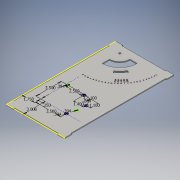
# Autodesk Inventor part: main board
Saved by Autodesk Inventor 2016 SP2 (Build 200236200, 236)
## iProperties
Created: 2017-09-03
Part Number: main board
Material: Generic
Document SubType Name: Modeling
Designer: Kartikye
Density: 1 g/cm^3
Appearance: Default
Author: Kartikye
Autodesk Inventor part; units mm, degrees
ref_plane "YZ Plane" through (0, 0, 0) normal (1, 0, 0) x (0, 1, 0)
ref_plane "XZ Plane" through (0, 0, 0) normal (0, 1, 0) x (-1, 0, 0)
ref_plane "XY Plane" through (0, 0, 0) normal (0, 0, 1) x (1, 0, 0)
sketch "Sketch1" plane through (0, 0, 0) normal (0, 1, 0) x (-1, 0, 0)
  line L0 (0, 0) -> (203.2, 0)
  line L1 (203.2, 0) -> (203.2, -381)
  line L2 (203.2, -381) -> (0, -381)
  line L3 (0, -381) -> (0, 0)
  dimension "d0" = 203.2
  dimension "d1" = 381
  constraints: 8 end point, 2 parallel, 1 horizontal, 1 perpendicular
  measures "d0" distance of L1.end L2.end
  measures "d1" distance of L0.end L1.end
extrude "Extrusion1" add sketch "Sketch1" along normal blind 3.175
sketch "Sketch2" plane through (0, 3.175, 0) normal (0, 1, 0) x (1, 0, 0)
  circle A0 centre (-158.75, 351.3667) radius 3.175
  line L0 (-203.2, 381) -> (-203.2, 0) projected
  line L1 (0, 381) -> (-203.2, 381) projected
  point P0 (0, 0)
  dimension "d4" = 6.35
  dimension "d5" = 44.45
  dimension "d6" = 29.6333
  constraints: 1 centre point
  measures "d4" diameter of A0
  measures "d5" distance from line of L0 A0.centre
  measures "d6" distance from line of L1 A0.centre
extrude "Extrusion2" cut sketch "Sketch2" against normal blind 3.175
sketch "Sketch3" plane through (0, 3.175, 0) normal (0, 1, 0) x (1, 0, 0)
  line L0 (-203.2, 381) -> (-203.2, 0) projected
  line L1 (0, 381) -> (-203.2, 381) projected
  line L2 (-203.2, 381) -> (0, 381) projected
  line L3 (-203.2, 0) -> (-203.2, 381) projected
  circle A0 centre (-158.75, 351.3667) radius 3.175 projected
  line L4 (-158.75, 351.3667) -> (-158.75, 197.5357) construction
  arc A1 (-158.75, 224.3667) -> (-31.75, 351.3667) centre (-158.75, 351.3667) ccw construction
  line L5 (-31.75, 351.3667) -> (-158.75, 351.3667) construction
  line L6 (-56.0048, 276.7179) -> (-158.75, 351.3667) construction
  line L7 (-77.7972, 253.5115) -> (-158.75, 351.3667) construction
  line L8 (-60.8948, 270.4138) -> (-158.75, 351.3667) construction
  line L9 (-66.171, 264.4292) -> (-158.75, 351.3667) construction
  line L10 (-71.8125, 258.7877) -> (-158.75, 351.3667) construction
  line L11 (-57.9661, 280.1712) -> (-65.672, 285.7698)
  line L12 (-65.672, 285.7698) -> (-67.5382, 283.2012)
  line L13 (-67.5382, 283.2012) -> (-59.8323, 277.6025)
  line L14 (-59.8323, 277.6025) -> (-57.9661, 280.1712)
  arc A2 (-77.7972, 253.5115) -> (-56.0048, 276.7179) centre (-158.75, 351.3667) ccw
  circle A3 centre (-67.9205, 285.3752) radius 1.27
  line L15 (-64.6418, 271.5575) -> (-62.6185, 274.0043)
  line L16 (-62.6185, 274.0043) -> (-69.959, 280.0742)
  line L17 (-71.9823, 277.6274) -> (-64.6418, 271.5575)
  line L18 (-69.959, 280.0742) -> (-71.9823, 277.6274)
  circle A4 centre (-72.2278, 279.8211) radius 1.27
  arc A5 (-166.6967, 224.6155) -> (-31.9989, 343.4199) centre (-158.75, 351.3667) ccw construction
  line L19 (-69.8201, 265.8253) -> (-67.6477, 268.1407)
  line L20 (-67.6477, 268.1407) -> (-74.5939, 274.658)
  line L21 (-76.7664, 272.3426) -> (-69.8201, 265.8253)
  line L22 (-74.5939, 274.658) -> (-76.7664, 272.3426)
  circle A6 centre (-76.8742, 274.5473) radius 1.27
  arc A7 (-174.6123, 225.3612) -> (-32.7445, 335.5043) centre (-158.75, 351.3667) ccw construction
  line L23 (-75.3469, 260.4283) -> (-73.0339, 262.6033)
  line L24 (-73.0339, 262.6033) -> (-79.5587, 269.5425)
  line L25 (-81.8718, 267.3675) -> (-75.3469, 260.4283)
  line L26 (-79.5587, 269.5425) -> (-81.8718, 267.3675)
  circle A8 centre (-81.8414, 269.5747) radius 1.27
  arc A9 (-182.4658, 226.6006) -> (-33.984, 327.6509) centre (-158.75, 351.3667) ccw construction
  line L27 (-81.2006, 255.3878) -> (-78.756, 257.4137)
  line L28 (-78.756, 257.4137) -> (-84.8339, 264.7476)
  line L29 (-87.2785, 262.7216) -> (-81.2006, 255.3878)
  line L30 (-84.8339, 264.7476) -> (-87.2785, 262.7216)
  circle A10 centre (-87.1101, 264.9226) radius 1.27
  arc A11 (-190.2263, 228.3291) -> (-35.7124, 319.8904) centre (-158.75, 351.3667) ccw construction
  line L31 (-28.9364, 348.5365) -> (-28.9236, 349.6672)
  line L32 (-28.9236, 349.6672) -> (-31.7607, 349.6994)
  line L33 (-31.7607, 349.6994) -> (-31.7555, 350.1627)
  line L34 (-31.7555, 350.1627) -> (-28.9183, 350.1305)
  line L35 (-28.9183, 350.1305) -> (-28.9056, 351.2481)
  line L36 (-28.9056, 351.2481) -> (-28.568, 351.2442)
  line L37 (-28.568, 351.2442) -> (-28.5988, 348.5327)
  line L38 (-28.5988, 348.5327) -> (-28.9364, 348.5365)
  line L39 (-32.0967, 341.9) -> (-32.0669, 342.3623)
  line L40 (-32.0669, 342.3623) -> (-30.6668, 342.272)
  line L41 (-30.6668, 342.272) -> (-30.5595, 343.9359)
  line L42 (-30.5595, 343.9359) -> (-31.9596, 344.0262)
  line L43 (-31.9596, 344.0262) -> (-31.9298, 344.4885)
  line L44 (-31.9298, 344.4885) -> (-28.7613, 344.2842)
  line L45 (-28.7613, 344.2842) -> (-28.7912, 343.8219)
  line L46 (-28.7912, 343.8219) -> (-30.2226, 343.9142)
  line L47 (-30.2226, 343.9142) -> (-30.3298, 342.2503)
  line L48 (-30.3298, 342.2503) -> (-28.8984, 342.158)
  line L49 (-28.8984, 342.158) -> (-28.9283, 341.6957)
  line L50 (-28.9283, 341.6957) -> (-32.0967, 341.9)
  spline S0 degree 2 poles (-32.0758, 334.4167) (-31.8629, 334.3895) (-31.53, 334.682) (-31.375, 335.0897) knots 0 0 0 1 2 2 2
  spline S1 degree 2 poles (-31.375, 335.0897) (-31.1895, 335.5911) (-30.653, 336.1136) (-30.3025, 336.0688) knots 0 0 0 1 2 2 2
  spline S2 degree 2 poles (-30.3025, 336.0688) (-29.9338, 336.0217) (-29.5205, 335.3329) (-29.5842, 334.8344) knots 0 0 0 1 2 2 2
  spline S3 degree 2 poles (-29.5842, 334.8344) (-29.6529, 334.297) (-30.2979, 333.7303) (-30.6731, 333.7888) knots 0 0 0 1 2 2 2
  line L51 (-30.6731, 333.7888) -> (-30.6854, 333.7957)
  line L52 (-30.6854, 333.7957) -> (-30.6293, 334.2344)
  spline S4 degree 2 poles (-30.6293, 334.2344) (-30.3619, 334.2003) (-29.9596, 334.5605) (-29.9191, 334.8772) knots 0 0 0 1 2 2 2
  spline S5 degree 2 poles (-29.9191, 334.8772) (-29.878, 335.1992) (-30.1224, 335.5787) (-30.356, 335.6086) knots 0 0 0 1 2 2 2
  spline S6 degree 2 poles (-30.356, 335.6086) (-30.5612, 335.6348) (-30.8819, 335.2932) (-31.0398, 334.8833) knots 0 0 0 1 2 2 2
  spline S7 degree 2 poles (-31.0398, 334.8833) (-31.2302, 334.3851) (-31.7792, 333.9091) (-32.1323, 333.9542) knots 0 0 0 1 2 2 2
  spline S8 degree 2 poles (-32.1323, 333.9542) (-32.5114, 334.0026) (-32.8905, 334.7108) (-32.8242, 335.2301) knots 0 0 0 1 2 2 2
  spline S9 degree 2 poles (-32.8242, 335.2301) (-32.7611, 335.7234) (-32.1557, 336.4139) (-31.7289, 336.3461) knots 0 0 0 1 2 2 2
  line L53 (-31.7289, 336.3461) -> (-31.7163, 336.3419)
  line L54 (-31.7163, 336.3419) -> (-31.7727, 335.9005)
  spline S10 degree 2 poles (-31.7727, 335.9005) (-32.0687, 335.9383) (-32.4527, 335.494) (-32.4918, 335.1876) knots 0 0 0 1 2 2 2
  spline S11 degree 2 poles (-32.4918, 335.1876) (-32.5337, 334.8605) (-32.3095, 334.4465) (-32.0758, 334.4167) knots 0 0 0 1 2 2 2
  line L55 (-32.4656, 327.2848) -> (-31.047, 326.1028)
  line L56 (-31.047, 326.1028) -> (-31.1465, 325.5809)
  line L57 (-31.1465, 325.5809) -> (-32.9418, 327.1491)
  line L58 (-32.9418, 327.1491) -> (-34.0397, 327.3585)
  line L59 (-34.0397, 327.3585) -> (-33.9534, 327.811)
  line L60 (-33.9534, 327.811) -> (-32.8247, 327.5957)
  line L61 (-32.8247, 327.5957) -> (-30.6125, 328.3809)
  line L62 (-30.6125, 328.3809) -> (-30.7115, 327.8615)
  line L63 (-30.7115, 327.8615) -> (-32.4656, 327.2848)
  line L64 (-34.3099, 320.2407) -> (-35.5423, 320.5558)
  line L65 (-35.5423, 320.5558) -> (-35.4275, 321.0046)
  line L66 (-35.4275, 321.0046) -> (-32.3515, 320.2182)
  line L67 (-32.3515, 320.2182) -> (-32.6763, 318.9477)
  spline S12 degree 2 poles (-32.6763, 318.9477) (-32.8125, 318.4151) (-33.4707, 317.9539) (-33.8841, 318.0596) knots 0 0 0 1 2 2 2
  spline S13 degree 2 poles (-33.8841, 318.0596) (-34.3025, 318.1666) (-34.6561, 318.8865) (-34.5199, 319.419) knots 0 0 0 1 2 2 2
  line L68 (-34.5199, 319.419) -> (-34.3099, 320.2407)
  line L69 (-33.9827, 320.157) -> (-34.1928, 319.3354)
  spline S14 degree 2 poles (-34.1928, 319.3354) (-34.279, 318.9981) (-34.0299, 318.5778) (-33.7737, 318.5123) knots 0 0 0 1 2 2 2
  spline S15 degree 2 poles (-33.7737, 318.5123) (-33.5176, 318.4468) (-33.0897, 318.694) (-33.0035, 319.0313) knots 0 0 0 1 2 2 2
  line L70 (-33.0035, 319.0313) -> (-32.7934, 319.8529)
  line L71 (-32.7934, 319.8529) -> (-33.9827, 320.157)
  spline S16 degree 2 poles (-37.1074, 310.5406) (-37.6602, 310.7196) (-38.1497, 311.6979) (-37.9578, 312.2906) knots 0 0 0 1 2 2 2
  spline S17 degree 2 poles (-37.9578, 312.2906) (-37.7732, 312.8608) (-36.8122, 313.3393) (-36.2593, 313.1604) knots 0 0 0 1 2 2 2
  line L72 (-36.2593, 313.1604) -> (-35.7214, 312.9862)
  spline S18 degree 2 poles (-35.7214, 312.9862) (-35.1711, 312.8081) (-34.6678, 311.8556) (-34.8525, 311.2853) knots 0 0 0 1 2 2 2
  spline S19 degree 2 poles (-34.8525, 311.2853) (-35.0443, 310.6926) (-36.0167, 310.1875) (-36.5695, 310.3665) knots 0 0 0 1 2 2 2
  line L73 (-36.5695, 310.3665) -> (-37.1074, 310.5406)
  spline S20 degree 2 poles (-36.421, 310.8082) (-36.0077, 310.6743) (-35.3208, 310.9857) (-35.1886, 311.3941) knots 0 0 0 1 2 2 2
  spline S21 degree 2 poles (-35.1886, 311.3941) (-35.0637, 311.7801) (-35.4458, 312.41) (-35.8592, 312.5439) knots 0 0 0 1 2 2 2
  line L74 (-35.8592, 312.5439) -> (-36.402, 312.7196)
  spline S22 degree 2 poles (-36.402, 312.7196) (-36.8204, 312.855) (-37.4991, 312.5685) (-37.6241, 312.1825) knots 0 0 0 1 2 2 2
  spline S23 degree 2 poles (-37.6241, 312.1825) (-37.7571, 311.7717) (-37.3848, 311.1201) (-36.9639, 310.9839) knots 0 0 0 1 2 2 2
  line L75 (-36.9639, 310.9839) -> (-36.421, 310.8082)
  line L76 (-39.9728, 302.4007) -> (-39.4456, 303.7065)
  line L77 (-39.4456, 303.7065) -> (-40.499, 304.1317)
  line L78 (-40.499, 304.1317) -> (-41.1163, 302.6026)
  line L79 (-41.1163, 302.6026) -> (-41.427, 302.7281)
  line L80 (-41.427, 302.7281) -> (-40.6363, 304.6868)
  line L81 (-40.6363, 304.6868) -> (-37.6921, 303.4982)
  line L82 (-37.6921, 303.4982) -> (-38.4731, 301.5638)
  line L83 (-38.4731, 301.5638) -> (-38.7862, 301.6902)
  line L84 (-38.7862, 301.6902) -> (-38.1787, 303.195)
  line L85 (-38.1787, 303.195) -> (-39.1325, 303.5801)
  line L86 (-39.1325, 303.5801) -> (-39.6597, 302.2743)
  line L87 (-39.6597, 302.2743) -> (-39.9728, 302.4007)
  line L88 (-42.5334, 296.8254) -> (-43.7767, 297.4169)
  line L89 (-43.7767, 297.4169) -> (-43.5777, 297.8352)
  line L90 (-43.5777, 297.8352) -> (-40.7129, 296.4725)
  line L91 (-40.7129, 296.4725) -> (-41.2166, 295.4136)
  spline S24 degree 2 poles (-41.2166, 295.4136) (-41.4583, 294.9054) (-42.1319, 294.5678) (-42.529, 294.7567) knots 0 0 0 1 2 2 2
  spline S25 degree 2 poles (-42.529, 294.7567) (-42.7489, 294.8613) (-42.957, 295.2646) (-42.9403, 295.5495) knots 0 0 0 1 2 2 2
  spline S26 degree 2 poles (-42.9403, 295.5495) (-43.1398, 295.3313) (-43.5882, 295.2721) (-43.8435, 295.3936) knots 0 0 0 1 2 2 2
  line L92 (-43.8435, 295.3936) -> (-44.1129, 295.5218)
  spline S27 degree 2 poles (-44.1129, 295.5218) (-44.2477, 295.5858) (-44.4908, 295.6232) (-44.5952, 295.5743) knots 0 0 0 1 2 2 2
  line L93 (-44.5952, 295.5743) -> (-44.6424, 295.5968)
  line L94 (-44.6424, 295.5968) -> (-44.4367, 296.0294)
  spline S28 degree 2 poles (-44.4367, 296.0294) (-44.3311, 296.0806) (-44.0487, 296.0042) (-43.9092, 295.9379) knots 0 0 0 1 2 2 2
  line L95 (-43.9092, 295.9379) -> (-43.6492, 295.8142)
  spline S29 degree 2 poles (-43.6492, 295.8142) (-43.4152, 295.7029) (-42.9921, 295.8611) (-42.8752, 296.1069) knots 0 0 0 1 2 2 2
  line L96 (-42.8752, 296.1069) -> (-42.5334, 296.8254)
  line L97 (-42.2285, 296.6804) -> (-42.5129, 296.0824)
  spline S30 degree 2 poles (-42.5129, 296.0824) (-42.6816, 295.7278) (-42.5806, 295.2943) (-42.3253, 295.1728) knots 0 0 0 1 2 2 2
  spline S31 degree 2 poles (-42.3253, 295.1728) (-42.0842, 295.0582) (-41.6721, 295.236) (-41.5192, 295.5575) knots 0 0 0 1 2 2 2
  line L98 (-41.5192, 295.5575) -> (-41.2144, 296.198)
  line L99 (-41.2144, 296.198) -> (-42.2285, 296.6804)
  line L100 (-47.0424, 290.2452) -> (-47.8506, 288.7808)
  line L101 (-47.8506, 288.7808) -> (-48.1439, 288.9427)
  line L102 (-48.1439, 288.9427) -> (-47.1119, 290.8127)
  line L103 (-47.1119, 290.8127) -> (-44.3321, 289.2786)
  line L104 (-44.3321, 289.2786) -> (-44.556, 288.873)
  line L105 (-44.556, 288.873) -> (-47.0424, 290.2452)
  spline S32 degree 2 poles (-51.1536, 281.4624) (-51.3657, 281.5971) (-51.6558, 281.9704) (-51.7289, 282.1874) knots 0 0 0 1 2 2 2
  line L106 (-51.7289, 282.1874) -> (-52.3914, 282.0034)
  line L107 (-52.3914, 282.0034) -> (-52.4567, 282.4231)
  line L108 (-52.4567, 282.4231) -> (-51.7863, 282.6145)
  spline S33 degree 2 poles (-51.7863, 282.6145) (-51.7797, 282.8056) (-51.656, 283.186) (-51.5396, 283.3694) knots 0 0 0 1 2 2 2
  spline S34 degree 2 poles (-51.5396, 283.3694) (-51.2183, 283.8754) (-50.1682, 284.0985) (-49.6776, 283.787) knots 0 0 0 1 2 2 2
  line L109 (-49.6776, 283.787) -> (-49.2003, 283.484)
  spline S35 degree 2 poles (-49.2003, 283.484) (-48.712, 283.1739) (-48.4628, 282.1258) (-48.7841, 281.6198) knots 0 0 0 1 2 2 2
  spline S36 degree 2 poles (-48.7841, 281.6198) (-49.118, 281.0939) (-50.1858, 280.8479) (-50.6763, 281.1594) knots 0 0 0 1 2 2 2
  line L110 (-50.6763, 281.1594) -> (-51.1536, 281.4624)
  spline S37 degree 2 poles (-50.4222, 281.5499) (-50.0554, 281.317) (-49.3125, 281.4468) (-49.0824, 281.8092) knots 0 0 0 1 2 2 2
  spline S38 degree 2 poles (-49.0824, 281.8092) (-48.8649, 282.1517) (-49.0775, 282.8572) (-49.4443, 283.0901) knots 0 0 0 1 2 2 2
  line L111 (-49.4443, 283.0901) -> (-49.926, 283.3959)
  spline S39 degree 2 poles (-49.926, 283.3959) (-50.2972, 283.6316) (-51.026, 283.5239) (-51.2435, 283.1814) knots 0 0 0 1 2 2 2
  spline S40 degree 2 poles (-51.2435, 283.1814) (-51.475, 282.8168) (-51.2773, 282.0929) (-50.9039, 281.8558) knots 0 0 0 1 2 2 2
  line L112 (-50.9039, 281.8558) -> (-50.4222, 281.5499)
  line L113 (-55.7542, 275.674) -> (-54.9953, 276.7177)
  line L114 (-54.9953, 276.7177) -> (-55.4757, 277.4456)
  line L115 (-55.4757, 277.4456) -> (-55.1971, 277.8288)
  line L116 (-55.1971, 277.8288) -> (-53.3557, 274.9624)
  line L117 (-53.3557, 274.9624) -> (-53.5897, 274.6406)
  line L118 (-53.5897, 274.6406) -> (-56.8703, 275.5276)
  line L119 (-56.8703, 275.5276) -> (-56.5917, 275.9108)
  line L120 (-56.5917, 275.9108) -> (-55.7542, 275.674)
  line L121 (-54.7817, 276.3973) -> (-55.3835, 275.5695)
  line L122 (-55.3835, 275.5695) -> (-53.9902, 275.1713)
  line L123 (-53.9902, 275.1713) -> (-53.981, 275.184)
  line L124 (-53.981, 275.184) -> (-54.7817, 276.3973)
  line L125 (-61.2151, 270.0279) -> (-60.9174, 270.3862)
  line L126 (-60.9174, 270.3862) -> (-58.4753, 268.3572)
  line L127 (-58.4753, 268.3572) -> (-58.773, 267.9989)
  line L128 (-58.773, 267.9989) -> (-61.2151, 270.0279)
  line L129 (-66.6794, 262.4131) -> (-66.6925, 262.4183)
  spline S41 degree 2 poles (-66.6925, 262.4183) (-67.023, 262.7202) (-66.9798, 263.6379) (-66.5858, 264.0543) knots 0 0 0 1 2 2 2
  spline S42 degree 2 poles (-66.5858, 264.0543) (-66.1863, 264.4763) (-65.1293, 264.485) (-64.7035, 264.082) knots 0 0 0 1 2 2 2
  line L130 (-64.7035, 264.082) -> (-64.2929, 263.6934)
  spline S43 degree 2 poles (-64.2929, 263.6934) (-63.867, 263.2904) (-63.8157, 262.2327) (-64.2151, 261.8107) knots 0 0 0 1 2 2 2
  spline S44 degree 2 poles (-64.2151, 261.8107) (-64.6163, 261.3867) (-65.504, 261.2827) (-65.8408, 261.6122) knots 0 0 0 1 2 2 2
  line L131 (-65.8408, 261.6122) -> (-65.8467, 261.625)
  line L132 (-65.8467, 261.625) -> (-65.5409, 261.9482)
  spline S45 degree 2 poles (-65.5409, 261.9482) (-65.2994, 261.7197) (-64.7266, 261.7614) (-64.4603, 262.0428) knots 0 0 0 1 2 2 2
  spline S46 degree 2 poles (-64.4603, 262.0428) (-64.1941, 262.3241) (-64.2957, 263.0582) (-64.6075, 263.3533) knots 0 0 0 1 2 2 2
  line L133 (-64.6075, 263.3533) -> (-65.022, 263.7455)
  spline S47 degree 2 poles (-65.022, 263.7455) (-65.3375, 264.0442) (-66.0761, 264.1053) (-66.3424, 263.824) knots 0 0 0 1 2 2 2
  spline S48 degree 2 poles (-66.3424, 263.824) (-66.6087, 263.5426) (-66.6207, 262.9702) (-66.3736, 262.7363) knots 0 0 0 1 2 2 2
  line L134 (-66.3736, 262.7363) -> (-66.6794, 262.4131)
  spline S49 degree 2 poles (-72.7661, 257.3144) (-72.7957, 257.5265) (-72.5551, 258.1552) (-72.2028, 258.4835) knots 0 0 0 1 2 2 2
  spline S50 degree 2 poles (-72.2028, 258.4835) (-71.7681, 258.8887) (-70.7033, 258.8865) (-70.3107, 258.4652) knots 0 0 0 1 2 2 2
  line L135 (-70.3107, 258.4652) -> (-69.8645, 257.9866)
  spline S51 degree 2 poles (-69.8645, 257.9866) (-69.4701, 257.5634) (-69.5215, 256.5207) (-69.9542, 256.1174) knots 0 0 0 1 2 2 2
  spline S52 degree 2 poles (-69.9542, 256.1174) (-70.3735, 255.7265) (-71.2417, 255.6866) (-71.534, 256.0117) knots 0 0 0 1 2 2 2
  line L136 (-71.534, 256.0117) -> (-71.5391, 256.0249)
  line L137 (-71.5391, 256.0249) -> (-71.2136, 256.3283)
  spline S53 degree 2 poles (-71.2136, 256.3283) (-71.0155, 256.1158) (-70.4563, 256.1109) (-70.1845, 256.3644) knots 0 0 0 1 2 2 2
  spline S54 degree 2 poles (-70.1845, 256.3644) (-69.8973, 256.6321) (-69.9162, 257.3587) (-70.2017, 257.6651) knots 0 0 0 1 2 2 2
  line L138 (-70.2017, 257.6651) -> (-70.6515, 258.1476)
  spline S55 degree 2 poles (-70.6515, 258.1476) (-70.9388, 258.4558) (-71.6833, 258.5097) (-71.9743, 258.2385) knots 0 0 0 1 2 2 2
  spline S56 degree 2 poles (-71.9743, 258.2385) (-72.1964, 258.0314) (-72.3569, 257.6815) (-72.3522, 257.5498) knots 0 0 0 1 2 2 2
  line L139 (-72.3522, 257.5498) -> (-71.865, 257.0271)
  line L140 (-71.865, 257.0271) -> (-71.2963, 257.5572)
  line L141 (-71.2963, 257.5572) -> (-71.0679, 257.3121)
  line L142 (-71.0679, 257.3121) -> (-71.9754, 256.4662)
  line L143 (-71.9754, 256.4662) -> (-72.7661, 257.3144)
  line L144 (-76.3224, 250.6123) -> (-76.6799, 250.3177)
  line L145 (-76.6799, 250.3177) -> (-78.1132, 252.0568)
  spline S57 degree 2 poles (-78.1132, 252.0568) (-78.3962, 252.4002) (-78.279, 253.1718) (-77.9215, 253.4664) knots 0 0 0 1 2 2 2
  spline S58 degree 2 poles (-77.9215, 253.4664) (-77.5559, 253.7677) (-76.831, 253.7647) (-76.5577, 253.4167) knots 0 0 0 1 2 2 2
  line L146 (-76.5577, 253.4167) -> (-76.5535, 253.4033)
  line L147 (-76.5535, 253.4033) -> (-76.8968, 253.1203)
  spline S59 degree 2 poles (-76.8968, 253.1203) (-77.0849, 253.3485) (-77.4963, 253.3826) (-77.7084, 253.2078) knots 0 0 0 1 2 2 2
  spline S60 degree 2 poles (-77.7084, 253.2078) (-77.9064, 253.0447) (-77.9388, 252.5737) (-77.7557, 252.3515) knots 0 0 0 1 2 2 2
  line L148 (-77.7557, 252.3515) -> (-76.3224, 250.6123)
  line L149 (-83.023, 248.0395) -> (-83.3131, 248.3434)
  line L150 (-83.3131, 248.3434) -> (-83.3274, 248.3363)
  line L151 (-83.3274, 248.3363) -> (-83.1461, 247.9507)
  line L152 (-83.1461, 247.9507) -> (-82.4261, 245.9141)
  line L153 (-82.4261, 245.9141) -> (-82.7955, 245.6477)
  line L154 (-82.7955, 245.6477) -> (-84.5049, 246.9709)
  line L155 (-84.5049, 246.9709) -> (-84.8202, 247.2695)
  line L156 (-84.8202, 247.2695) -> (-84.8308, 247.2618)
  line L157 (-84.8308, 247.2618) -> (-84.6322, 246.879)
  line L158 (-84.6322, 246.879) -> (-83.8189, 244.9098)
  line L159 (-83.8189, 244.9098) -> (-84.2265, 244.6158)
  line L160 (-84.2265, 244.6158) -> (-85.4105, 247.6764)
  line L161 (-85.4105, 247.6764) -> (-85.0751, 247.9183)
  line L162 (-85.0751, 247.9183) -> (-83.2313, 246.5339)
  line L163 (-83.2313, 246.5339) -> (-83.022, 246.3331)
  line L164 (-83.022, 246.3331) -> (-83.0114, 246.3408)
  line L165 (-83.0114, 246.3408) -> (-83.1379, 246.6013)
  line L166 (-83.1379, 246.6013) -> (-83.8628, 248.7925)
  line L167 (-83.8628, 248.7925) -> (-83.5253, 249.0359)
  line L168 (-83.5253, 249.0359) -> (-80.9973, 246.9444)
  line L169 (-80.9973, 246.9444) -> (-81.4049, 246.6505)
  line L170 (-81.4049, 246.6505) -> (-83.023, 248.0395)
  line L171 (-89.8994, 240.8822) -> (-91.033, 242.6615)
  spline S61 degree 2 poles (-91.033, 242.6615) (-91.3143, 243.103) (-91.0112, 243.9913) (-90.5211, 244.3035) knots 0 0 0 1 2 2 2
  spline S62 degree 2 poles (-90.5211, 244.3035) (-90.0509, 244.6031) (-89.134, 244.4889) (-88.8542, 244.0496) knots 0 0 0 1 2 2 2
  line L172 (-88.8542, 244.0496) -> (-87.7206, 242.2703)
  line L173 (-87.7206, 242.2703) -> (-88.1135, 242.02)
  line L174 (-88.1135, 242.02) -> (-89.2471, 243.7993)
  spline S63 degree 2 poles (-89.2471, 243.7993) (-89.4426, 244.1061) (-90.0409, 244.2122) (-90.3411, 244.0209) knots 0 0 0 1 2 2 2
  spline S64 degree 2 poles (-90.3411, 244.0209) (-90.659, 243.8184) (-90.8378, 243.2173) (-90.6423, 242.9104) knots 0 0 0 1 2 2 2
  line L175 (-90.6423, 242.9104) -> (-89.5087, 241.1312)
  line L176 (-89.5087, 241.1312) -> (-89.8994, 240.8822)
  line L177 (-96.3627, 240.7396) -> (-94.83, 237.9591)
  line L178 (-94.83, 237.9591) -> (-95.7744, 237.4385)
  spline S65 degree 2 poles (-95.7744, 237.4385) (-96.3635, 237.1138) (-97.4489, 237.3912) (-97.7408, 237.9207) knots 0 0 0 1 2 2 2
  line L179 (-97.7408, 237.9207) -> (-97.9506, 238.3012)
  spline S66 degree 2 poles (-97.9506, 238.3012) (-98.2437, 238.833) (-97.8962, 239.8943) (-97.3071, 240.2191) knots 0 0 0 1 2 2 2
  line L180 (-97.3071, 240.2191) -> (-96.3627, 240.7396)
  line L181 (-95.3987, 238.0311) -> (-96.6067, 240.2226)
  line L182 (-96.6067, 240.2226) -> (-97.1453, 239.9256)
  spline S67 degree 2 poles (-97.1453, 239.9256) (-97.5625, 239.6957) (-97.7634, 238.9214) (-97.5448, 238.5249) knots 0 0 0 1 2 2 2
  line L183 (-97.5448, 238.5249) -> (-97.3325, 238.1398)
  spline S68 degree 2 poles (-97.3325, 238.1398) (-97.1165, 237.7478) (-96.3546, 237.5042) (-95.9374, 237.7342) knots 0 0 0 1 2 2 2
  line L184 (-95.9374, 237.7342) -> (-95.3987, 238.0311)
  line L185 (-103.5851, 235.3824) -> (-103.3129, 235.5109)
  line L186 (-103.3129, 235.5109) -> (-103.9253, 236.808)
  line L187 (-103.9253, 236.808) -> (-103.5063, 237.0058)
  line L188 (-103.5063, 237.0058) -> (-102.1508, 234.1347)
  line L189 (-102.1508, 234.1347) -> (-102.5698, 233.9369)
  line L190 (-102.5698, 233.9369) -> (-103.1698, 235.2079)
  line L191 (-103.1698, 235.2079) -> (-103.3994, 235.0995)
  line L192 (-103.3994, 235.0995) -> (-103.9497, 233.2854)
  line L193 (-103.9497, 233.2854) -> (-104.4231, 233.0619)
  line L194 (-104.4231, 233.0619) -> (-104.4323, 233.0691)
  line L195 (-104.4323, 233.0691) -> (-103.8169, 235.0211)
  line L196 (-103.8169, 235.0211) -> (-105.8688, 235.8788)
  line L197 (-105.8688, 235.8788) -> (-105.8685, 235.8905)
  line L198 (-105.8685, 235.8905) -> (-105.3596, 236.1308)
  line L199 (-105.3596, 236.1308) -> (-103.5851, 235.3824)
  line L200 (-111.0187, 231.59) -> (-111.3044, 230.1433)
  line L201 (-111.3044, 230.1433) -> (-111.8247, 229.936)
  line L202 (-111.8247, 229.936) -> (-111.3966, 231.8028)
  line L203 (-111.3966, 231.8028) -> (-113.0221, 232.8766)
  line L204 (-113.0221, 232.8766) -> (-112.509, 233.0811)
  line L205 (-112.509, 233.0811) -> (-111.2794, 232.2158)
  line L206 (-111.2794, 232.2158) -> (-110.9797, 233.6906)
  line L207 (-110.9797, 233.6906) -> (-110.4569, 233.899)
  line L208 (-110.4569, 233.899) -> (-110.8981, 232.0015)
  line L209 (-110.8981, 232.0015) -> (-109.3033, 230.9409)
  line L210 (-109.3033, 230.9409) -> (-109.8212, 230.7345)
  line L211 (-109.8212, 230.7345) -> (-111.0187, 231.59)
  line L212 (-118.0337, 231.0651) -> (-117.0427, 228.0487)
  line L213 (-117.0427, 228.0487) -> (-118.1045, 227.6999)
  spline S69 degree 2 poles (-118.1045, 227.6999) (-118.6168, 227.5316) (-119.3277, 227.7499) (-119.4617, 228.1577) knots 0 0 0 1 2 2 2
  spline S70 degree 2 poles (-119.4617, 228.1577) (-119.5262, 228.3541) (-119.3664, 228.7483) (-119.1787, 228.8981) knots 0 0 0 1 2 2 2
  spline S71 degree 2 poles (-119.1787, 228.8981) (-119.5134, 228.835) (-120.0277, 229.1426) (-120.1241, 229.4361) knots 0 0 0 1 2 2 2
  spline S72 degree 2 poles (-120.1241, 229.4361) (-120.2597, 229.8488) (-119.8216, 230.4777) (-119.3243, 230.6411) knots 0 0 0 1 2 2 2
  line L214 (-119.3243, 230.6411) -> (-118.0337, 231.0651)
  line L215 (-118.009, 229.5056) -> (-118.3693, 230.6022)
  line L216 (-118.3693, 230.6022) -> (-119.2197, 230.3228)
  spline S73 degree 2 poles (-119.2197, 230.3228) (-119.5231, 230.2231) (-119.7656, 229.8376) (-119.6823, 229.584) knots 0 0 0 1 2 2 2
  spline S74 degree 2 poles (-119.6823, 229.584) (-119.5998, 229.3328) (-119.1586, 229.1389) (-118.8669, 229.2237) knots 0 0 0 1 2 2 2
  line L217 (-118.8669, 229.2237) -> (-118.837, 229.2335)
  line L218 (-118.837, 229.2335) -> (-118.009, 229.5056)
  line L219 (-117.9044, 229.1873) -> (-118.6181, 228.9528)
  spline S75 degree 2 poles (-118.6181, 228.9528) (-118.8643, 228.8719) (-119.0926, 228.5186) (-119.0191, 228.2948) knots 0 0 0 1 2 2 2
  spline S76 degree 2 poles (-119.0191, 228.2948) (-118.939, 228.0511) (-118.5232, 227.9177) (-118.2099, 228.0207) knots 0 0 0 1 2 2 2
  line L220 (-118.2099, 228.0207) -> (-117.5882, 228.2249)
  line L221 (-117.5882, 228.2249) -> (-117.9044, 229.1873)
  line L222 (-128.0625, 228.1232) -> (-127.6141, 228.2397)
  line L223 (-127.6141, 228.2397) -> (-125.406, 226.3092)
  line L224 (-125.406, 226.3092) -> (-125.3914, 226.3157)
  line L225 (-125.3914, 226.3157) -> (-126.0004, 228.659)
  line L226 (-126.0004, 228.659) -> (-125.552, 228.7756)
  line L227 (-125.552, 228.7756) -> (-124.7534, 225.7026)
  line L228 (-124.7534, 225.7026) -> (-125.2018, 225.5861)
  line L229 (-125.2018, 225.5861) -> (-127.41, 227.5166)
  line L230 (-127.41, 227.5166) -> (-127.4239, 227.5076)
  line L231 (-127.4239, 227.5076) -> (-126.8156, 225.1668)
  line L232 (-126.8156, 225.1668) -> (-127.264, 225.0502)
  line L233 (-127.264, 225.0502) -> (-128.0625, 228.1232)
  line L234 (-135.1285, 225.1513) -> (-133.7078, 225.4285)
  line L235 (-133.7078, 225.4285) -> (-133.9765, 226.8055)
  line L236 (-133.9765, 226.8055) -> (-133.5217, 226.8942)
  line L237 (-133.5217, 226.8942) -> (-132.9139, 223.7779)
  line L238 (-132.9139, 223.7779) -> (-135.0256, 223.366)
  line L239 (-135.0256, 223.366) -> (-135.0903, 223.6974)
  line L240 (-135.0903, 223.6974) -> (-133.4332, 224.0206)
  line L241 (-133.4332, 224.0206) -> (-133.6427, 225.0945)
  line L242 (-133.6427, 225.0945) -> (-135.0634, 224.8174)
  line L243 (-135.0634, 224.8174) -> (-135.1285, 225.1513)
  line L244 (-142.4802, 224.8141) -> (-142.4931, 224.8124)
  line L245 (-142.4931, 224.8124) -> (-143.2517, 222.1127)
  line L246 (-143.2517, 222.1127) -> (-143.8228, 222.0393)
  line L247 (-143.8228, 222.0393) -> (-144.2278, 225.1883)
  line L248 (-144.2278, 225.1883) -> (-143.7683, 225.2474)
  line L249 (-143.7683, 225.2474) -> (-143.4648, 222.8876)
  line L250 (-143.4648, 222.8876) -> (-143.4489, 222.887)
  line L251 (-143.4489, 222.887) -> (-142.7247, 225.3817)
  line L252 (-142.7247, 225.3817) -> (-142.4028, 225.4231)
  line L253 (-142.4028, 225.4231) -> (-141.0297, 223.119)
  line L254 (-141.0297, 223.119) -> (-141.0145, 223.1236)
  line L255 (-141.0145, 223.1236) -> (-141.328, 225.5613)
  line L256 (-141.328, 225.5613) -> (-140.8685, 225.6204)
  line L257 (-140.8685, 225.6204) -> (-140.4635, 222.4713)
  line L258 (-140.4635, 222.4713) -> (-141.0684, 222.3935)
  line L259 (-141.0684, 222.3935) -> (-142.4802, 224.8141)
  line L260 (-150.7915, 223.7823) -> (-150.8835, 224.0414)
  line L261 (-150.8835, 224.0414) -> (-150.8992, 224.0405)
  line L262 (-150.8992, 224.0405) -> (-150.9613, 223.7718)
  line L263 (-150.9613, 223.7718) -> (-151.7, 221.3791)
  line L264 (-151.7, 221.3791) -> (-152.2016, 221.3481)
  line L265 (-152.2016, 221.3481) -> (-151.1249, 224.5956)
  line L266 (-151.1249, 224.5956) -> (-150.7278, 224.6201)
  line L267 (-150.7278, 224.6201) -> (-149.2599, 221.5297)
  line L268 (-149.2599, 221.5297) -> (-149.7615, 221.4987)
  line L269 (-149.7615, 221.4987) -> (-150.7915, 223.7823)
  line L270 (-157.9909, 224.032) -> (-159.9095, 224.031)
  line L271 (-159.9095, 224.031) -> (-159.9096, 224.366)
  line L272 (-159.9096, 224.366) -> (-157.4675, 224.3673)
  line L273 (-157.4675, 224.3673) -> (-157.4674, 224.048)
  line L274 (-157.4674, 224.048) -> (-159.2983, 221.529)
  line L275 (-159.2983, 221.529) -> (-157.4922, 221.53)
  line L276 (-157.4922, 221.53) -> (-157.492, 221.1923)
  line L277 (-157.492, 221.1923) -> (-159.8294, 221.1911)
  line L278 (-159.8294, 221.1911) -> (-159.8296, 221.4999)
  line L279 (-159.8296, 221.4999) -> (-157.9909, 224.032)
  point P0 (0, 0)
  point P1 (-54.3056, 381)
  point P2 (-203.2, 226.9326)
  point P3 (-32.0006, 343.3923)
  point P4 (-32.7514, 335.4493)
  point P5 (-33.9995, 327.5692)
  point P6 (-35.7399, 319.7831)
  point P7 (-37.9658, 312.1215)
  point P8 (-40.6684, 304.6148)
  point P9 (-43.837, 297.2927)
  point P10 (-47.4591, 290.184)
  point P11 (-51.5204, 283.3167)
  point P12 (-84.1013, 248.6215)
  point P13 (-90.7, 244.137)
  point P14 (-97.5673, 240.0757)
  point P15 (-104.676, 236.4536)
  point P16 (-111.9982, 233.2851)
  point P17 (-119.5048, 230.5825)
  point P18 (-127.1664, 228.3566)
  point P19 (-134.9526, 226.6162)
  point P20 (-142.8327, 225.3681)
  point P21 (-150.7756, 224.6173)
  point P22 (-158.75, 224.3667)
  dimension "d15" = 90
  dimension "d17" = 0
  dimension "d18" = 0
  dimension "d19" = 9.525
  dimension "d20" = 3.175
  dimension "d25" = 2.54
  dimension "d28" = 14.35
  constraints: 54 end point, 13 point on circle, 11 centre point, 4 point on line, 2 parallel, 1 perpendicular, 1 vertical, 84 other
  measures "d17" distance of A0.centre L5.end
  measures "d18" distance from line of A0.centre L5
  measures "d19" distance of L13.end L12.end
  measures "d20" distance of L12.end L11.end
  measures "d25" diameter of A3
sketch "Sketch5" plane through (0, 3.175, 0) normal (0, 1, 0) x (1, 0, 0)
  line L0 (-203.2, 381) -> (-203.2, 0)
  line L1 (0, 381) -> (-203.2, 381)
  line L2 (-203.2, 381) -> (0, 381)
  line L3 (-203.2, 0) -> (-203.2, 381)
  circle A0 centre (-158.75, 351.3667) radius 3.175
  line L4 (-158.75, 351.3667) -> (-158.75, 197.5357) construction
  arc A1 (-158.75, 224.3667) -> (-31.75, 351.3667) centre (-158.75, 351.3667) ccw construction
  line L5 (-31.75, 351.3667) -> (-158.75, 351.3667) construction
  line L6 (-56.0048, 276.7179) -> (-158.75, 351.3667) construction
  line L7 (-77.7972, 253.5115) -> (-158.75, 351.3667) construction
  line L8 (-60.8948, 270.4138) -> (-158.75, 351.3667) construction
  line L9 (-66.171, 264.4292) -> (-158.75, 351.3667) construction
  line L10 (-71.8125, 258.7877) -> (-158.75, 351.3667) construction
  line L11 (-57.9661, 280.1712) -> (-65.672, 285.7698)
  line L12 (-65.672, 285.7698) -> (-67.5382, 283.2012)
  line L13 (-67.5382, 283.2012) -> (-59.8323, 277.6025)
  line L14 (-59.8323, 277.6025) -> (-57.9661, 280.1712)
  arc A2 (-77.7972, 253.5115) -> (-56.0048, 276.7179) centre (-158.75, 351.3667) ccw
  circle A3 centre (-67.9205, 285.3752) radius 1.27
  line L15 (-64.6418, 271.5575) -> (-62.6185, 274.0043)
  line L16 (-62.6185, 274.0043) -> (-69.959, 280.0742)
  line L17 (-71.9823, 277.6274) -> (-64.6418, 271.5575)
  line L18 (-69.959, 280.0742) -> (-71.9823, 277.6274)
  circle A4 centre (-72.2278, 279.8211) radius 1.27
  arc A5 (-166.6967, 224.6155) -> (-31.9989, 343.4199) centre (-158.75, 351.3667) ccw construction
  line L19 (-69.8201, 265.8253) -> (-67.6477, 268.1407)
  line L20 (-67.6477, 268.1407) -> (-74.5939, 274.658)
  line L21 (-76.7664, 272.3426) -> (-69.8201, 265.8253)
  line L22 (-74.5939, 274.658) -> (-76.7664, 272.3426)
  circle A6 centre (-76.8742, 274.5473) radius 1.27
  arc A7 (-174.6123, 225.3612) -> (-32.7445, 335.5043) centre (-158.75, 351.3667) ccw construction
  line L23 (-75.3469, 260.4283) -> (-73.0339, 262.6033)
  line L24 (-73.0339, 262.6033) -> (-79.5587, 269.5425)
  line L25 (-81.8718, 267.3675) -> (-75.3469, 260.4283)
  line L26 (-79.5587, 269.5425) -> (-81.8718, 267.3675)
  circle A8 centre (-81.8414, 269.5747) radius 1.27
  arc A9 (-182.4658, 226.6006) -> (-33.984, 327.6509) centre (-158.75, 351.3667) ccw construction
  line L27 (-81.2006, 255.3878) -> (-78.756, 257.4137)
  line L28 (-78.756, 257.4137) -> (-84.8339, 264.7476)
  line L29 (-87.2785, 262.7216) -> (-81.2006, 255.3878)
  line L30 (-84.8339, 264.7476) -> (-87.2785, 262.7216)
  circle A10 centre (-87.1101, 264.9226) radius 1.27
  arc A11 (-190.2263, 228.3291) -> (-35.7124, 319.8904) centre (-158.75, 351.3667) ccw construction
  point P0 (0, 0)
  point P1 (-54.3056, 381)
  point P2 (-203.2, 226.9326)
  point P3 (-32.0006, 343.3923)
  point P4 (-32.7514, 335.4493)
  point P5 (-33.9995, 327.5692)
  point P6 (-35.7399, 319.7831)
  point P7 (-37.9658, 312.1215)
  point P8 (-40.6684, 304.6148)
  point P9 (-43.837, 297.2927)
  point P10 (-47.4591, 290.184)
  point P11 (-51.5204, 283.3167)
  point P12 (-84.1013, 248.6215)
  point P13 (-90.7, 244.137)
  point P14 (-97.5673, 240.0757)
  point P15 (-104.676, 236.4536)
  point P16 (-111.9982, 233.2851)
  point P17 (-119.5048, 230.5825)
  point P18 (-127.1664, 228.3566)
  point P19 (-134.9526, 226.6162)
  point P20 (-142.8327, 225.3681)
  point P21 (-150.7756, 224.6173)
  point P22 (-158.75, 224.3667)
  dimension "d34" = 90
  dimension "d35" = 0
  dimension "d36" = 0
  dimension "d37" = 9.525
  dimension "d38" = 3.175
  dimension "d39" = 2.54
  dimension "d40" = 14.35
  constraints: 62 end point, 13 point on circle, 12 centre point, 4 point on line, 2 parallel, 1 perpendicular, 1 vertical, 84 other
  measures "d35" distance of A0.centre L7.end
  measures "d36" distance from line of A0.centre L5
  measures "d37" distance of L14.start L12.end
  measures "d38" distance of L12.end L12.start
  measures "d39" diameter of A3
extrude "Extrusion3" cut sketch "Sketch5" against normal blind 3.175 contours L14 L13 L12 L11 | A3 | L17 L18 L16 L15 | A4 | L21 L22 L20 L19 | A6 | L25 L26 L24 L23 | A8 | L29 L30 L28 L27 | A10
extrude "Extrusion4" cut sketch "Sketch3" against normal blind 3.175 contours A2 L126 L127 L128 | S49 S50 A2 | A2 S50 L135 S51 S52 L136 L137 S53 S54 L138 S55 S56 L139 L140 L141 L142 L143 S49 | S41 S42 A2 | A2 S42 L130 S43 S44 L131 L132 S45 S46 L133 S47 S48 L134 L129 S41 | L31 L32 L33 L34 L35 L36 L37 L38 | L39 L40 L41 L42 L43 L44 L45 L46 L47 L48 L49 L50 | S0 S1 S2 S3 L51 L52 S4 S5 S6 S7 S8 S9 L53 L54 S10 S11 | L55 L56 L57 L58 L59 L60 L61 L62 L63 | L64 L65 L66 L67 S12 S13 L68 | S16 S17 L72 S18 S19 L73 | L76 L77 L78 L79 L80 L81 L82 L83 L84 L85 L86 L87 | L88 L89 L90 L91 S24 S25 S26 L92 S27 L93 L94 S28 L95 S29 L96 | L100 L101 L102 L103 L104 L105 | S32 L106 L107 L108 S33 S34 L109 S35 S36 L110 | L113 L114 L115 L116 L117 L118 L119 L120 | L144 L145 S57 S58 L146 L147 S59 S60 L148 | L149 L150 L151 L152 L153 L154 L155 L156 L157 L158 L159 L160 L161 L162 L163 L164 L165 L166 L167 L168 L169 L170 | L171 S61 S62 L172 L173 L174 S63 S64 L175 L176 | L177 L178 S65 L179 S66 L180 | L185 L186 L187 L188 L189 L190 L191 L192 L193 L194 L195 L196 L197 L198 L199 | L200 L201 L202 L203 L204 L205 L206 L207 L208 L209 L210 L211 | L212 L213 S69 S70 S71 S72 L214 | L222 L223 L224 L225 L226 L227 L228 L229 L230 L231 L232 L233 | L234 L235 L236 L237 L238 L239 L240 L241 L242 L243 | L244 L245 L246 L247 L248 L249 L250 L251 L252 L253 L254 L255 L256 L257 L258 L259 | L260 L261 L262 L263 L264 L265 L266 L267 L268 L269 | L270 L271 L272 L273 L274 L275 L276 L277 L278 L279
sketch "Sketch6" plane through (0, 3.175, 0) normal (0, 1, 0) x (1, 0, 0)
  circle A0 centre (-158.75, 351.3667) radius 3.175 projected
  line L0 (-158.75, 351.3667) -> (-14.3792, 351.3667) construction
  line L1 (-158.75, 351.3667) -> (-158.75, 192.8963) construction
  arc A1 (-158.75, 315.8067) -> (-123.19, 351.3667) centre (-158.75, 351.3667) ccw
  arc A2 (-158.75, 290.4067) -> (-97.79, 351.3667) centre (-158.75, 351.3667) ccw
  line L2 (-97.79, 351.3667) -> (-123.19, 351.3667)
  line L3 (-158.75, 315.8067) -> (-158.75, 290.4067)
  point P0 (0, 0)
  dimension "d45" = 35.56
  dimension "d46" = 35.56
  dimension "d47" = 60.96
  dimension "d48" = 60.96
  constraints: 8 end point, 5 point on circle, 4 point on line, 2 centre point, 1 collinear, 1 concentric, 1 horizontal, 1 vertical
  measures "d45" distance of L0.start L2.end
  measures "d46" distance of L3.start L0.start
  measures "d47" distance of L2.start L0.start
  measures "d48" distance of A2.start L0.start
extrude "Extrusion5" cut sketch "Sketch6" against normal blind 3.175 contours A1 L2 A2 L3
sketch "Sketch7" plane through (0, 3.175, 0) normal (0, 1, 0) x (1, 0, 0)
  circle A0 centre (-158.75, 76.2) radius 3.175 construction
  line L0 (-203.2, 381) -> (-203.2, 0) projected
  line L1 (-203.2, 0) -> (0, 0) projected
  line L2 (-158.75, 76.2) -> (-21.2116, 76.2) construction
  line L3 (-158.75, 76.2) -> (-158.75, 211.0379) construction
  circle A1 centre (-153.6277, 165.1) radius 5
  circle A2 centre (-95.25, 162.56) radius 5
  circle A3 centre (-59.69, 134.62) radius 5
  circle A4 centre (-62.166, 103.0071) radius 5
  circle A5 centre (-69.85, 76.2) radius 5
  point P0 (-158.75, 165.1)
  dimension "d51" = 6.35
  dimension "d52" = 44.45
  dimension "d53" = 76.2
  dimension "d54" = 88.9
  dimension "d55" = 88.9
  dimension "d57" = 2.54
  dimension "d58" = 63.5
  dimension "d59" = 35.56
  dimension "d60" = 27.94
  dimension "d61" = 10
  dimension "d62" = 10
  dimension "d63" = 10
  dimension "d64" = 10
  dimension "d65" = 10
  constraints: 6 centre point, 4 coincident, 4 end point, 2 point on line, 1 horizontal, 1 vertical
  measures "d51" diameter of A0
  measures "d52" distance from line of L0 L2.start
  measures "d53" distance from line of L2.start L1
  measures "d54" distance of L2.start point (-158.75, 165.1)
  measures "d55" distance of point (-69.85, 76.2) L2.start
  measures "d57" vertical distance of point (-95.25, 162.56) point (-158.75, 165.1)
  measures "d58" horizontal distance of point (-158.75, 165.1) point (-95.25, 162.56)
  measures "d59" horizontal distance of point (-59.69, 134.62) point (-95.25, 162.56)
  measures "d60" vertical distance of point (-59.69, 134.62) point (-95.25, 162.56)
  measures "d61" diameter of A1
  measures "d62" diameter of A2
  measures "d63" diameter of A3
  measures "d64" diameter of A4
  measures "d65" diameter of A5
sketch "Sketch8" plane through (0, 3.175, 0) normal (0, 1, 0) x (1, 0, 0)
  line L0 (0, 25.4) -> (-3.175, 25.4)
  line L1 (-3.175, 25.4) -> (-3.175, 355.6)
  line L2 (-3.175, 355.6) -> (0, 355.6)
  line L3 (0, 381) -> (0, 0) projected
  line L4 (0, 25.4) -> (75.5054, 210.8617)
  line L5 (75.5054, 210.8617) -> (0, 355.6)
  line L6 (0, 0) -> (-17.4749, 17.4749) construction
  line L7 (0, 0) -> (24.7133, 0) construction
  line L8 (-25.4, 0) -> (-25.4, 3.175)
  line L9 (-203.2, 381) -> (0, 381) projected
  line L10 (-101.6, 381) -> (-101.6, 279.1154) construction
  line L11 (-203.2, 25.4) -> (-200.025, 25.4)
  line L12 (-200.025, 25.4) -> (-200.025, 355.6)
  line L13 (-200.025, 355.6) -> (-203.2, 355.6)
  line L14 (-203.2, 25.4) -> (-278.7054, 210.8617)
  line L15 (-278.7054, 210.8617) -> (-203.2, 355.6)
  line L16 (-203.2, 0) -> (-185.7251, 17.4749) construction
  line L17 (-177.8, 0) -> (-177.8, 3.175)
  line L18 (-25.4, 3.175) -> (-177.8, 3.175)
  line L19 (-203.2, 0) -> (0, 0) projected
  line L20 (-177.8, 0) -> (-66.857, -66.857)
  line L21 (-66.857, -66.857) -> (-25.4, 0)
  line L22 (-203.2, 0) -> (-203.2, 381) projected
  line L23 (-203.2, 190.5) -> (-124.6961, 190.5) construction
  line L24 (-25.4, 381) -> (-25.4, 377.825)
  line L25 (-177.8, 381) -> (-177.8, 377.825)
  line L26 (-25.4, 377.825) -> (-177.8, 377.825)
  line L27 (-177.8, 381) -> (-66.857, 447.857)
  line L28 (-66.857, 447.857) -> (-25.4, 381)
  point P0 (-25.4, 0)
  dimension "d66" = 25.4
  dimension "d67" = 25.4
  dimension "d68" = 3.175
  dimension "d69" = 330.2
  dimension "d70" = 90
  dimension "d71" = 135
  constraints: 50 end point, 16 symmetric about line, 3 horizontal, 2 midpoint, 2 perpendicular, 1 equal length, 1 parallel, 1 point on line, 1 vertical
  measures "d66" distance of L3.end L0.start
  measures "d67" distance of L3.end point (-25.4, 0)
  measures "d68" distance of L0.start L0.end
  measures "d69" distance of L0.end L1.end
  measures "d70" angle of L0 L1
  measures "d71" angle of L7 L6
extrude "Extrusion6" cut sketch "Sketch8" against normal blind 3.175 contours L0 L1 L2 L3 | L3 L5 L4 | L19 L17 L18 L8 | L21 L20 L19 | L24 L26 L25 L9 | L9 L27 L28 | L22 L13 L12 L11 | L14 L15 L22
sketch "Sketch9" plane through (0, 3.175, 0) normal (0, 1, 0) x (1, 0, 0)
  point P0 (0, 0)
sketch "Sketch10" plane through (0, 3.175, 0) normal (0, 1, 0) x (1, 0, 0)
  circle A0 centre (-158.75, 351.3667) radius 3.175 projected
  line L0 (-158.75, 351.3667) -> (-158.75, 239.7125) construction
  arc A1 (-158.75, 275.1667) -> (-82.55, 351.3667) centre (-158.75, 351.3667) ccw
  arc A2 (-158.75, 267.5467) -> (-74.93, 351.3667) centre (-158.75, 351.3667) ccw
  line L1 (-158.75, 351.3667) -> (-52.3875, 289.9582)
  line L2 (-158.75, 351.3667) -> (-35.9332, 351.3667) construction
  line L3 (-158.75, 351.3667) -> (-95.2893, 257.2823)
  point P0 (0, 0)
  point P1 (-86.1598, 309.4567)
  point P2 (-92.7589, 313.2667)
  point P3 (-111.8785, 281.8767)
  point P4 (-116.1395, 288.194)
  dimension "d74" = 76.2
  dimension "d75" = 76.2
  dimension "d76" = 76.2
  dimension "d77" = 7.62
  dimension "d78" = 7.62
  dimension "d79" = 30
  dimension "d80" = 34
  constraints: 8 end point, 8 point on circle, 6 point on line, 2 centre point, 1 equal length, 1 horizontal, 1 vertical
  measures "d74" distance of L0.start A1.end
  measures "d75" distance of A1.start L0.start
  measures "d76" radius of A1
  measures "d77" distance of A1.end A2.end
  measures "d78" distance of A1.start A2.start
  measures "d79" angle of L1 L2
  measures "d80" angle of L0 L3
extrude "Extrusion7" cut sketch "Sketch10" against normal blind 3.175 contours A1 L1 A2 L3
body "Solid1"
